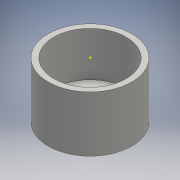
# Autodesk Inventor part: motor_hinge_cup
Saved by Autodesk Inventor 2016 (Build 200138000, 138)
## iProperties
Created: 2016-11-10
Part Number: motor_hinge_cup
Material: Generic
Document SubType Name: Modeling
Designer: Sa'id
Density: 1 g/cm^3
Appearance: Default
Author: Sa'id
Autodesk Inventor part; units mm, degrees
ref_plane "YZ Plane" through (0, 0, 0) normal (1, 0, 0) x (0, 1, 0)
ref_plane "XZ Plane" through (0, 0, 0) normal (0, 1, 0) x (-1, 0, 0)
ref_plane "XY Plane" through (0, 0, 0) normal (0, 0, 1) x (1, 0, 0)
sketch "Sketch1" plane through (0, 0, 0) normal (0, 0, 1) x (1, 0, 0)
  circle A0 centre (0, 0) radius 3.75
  dimension "d0" = 7.5
  constraints: 1 centre point, 1 coincident
  measures "d0" diameter of A0
extrude "Extrusion1" add sketch "Sketch1" along normal blind 5
hole "Hole1" at (0, 0, 5) direction (0, 0, -1) diameter 6.5 depth 4
body "Solid1"
